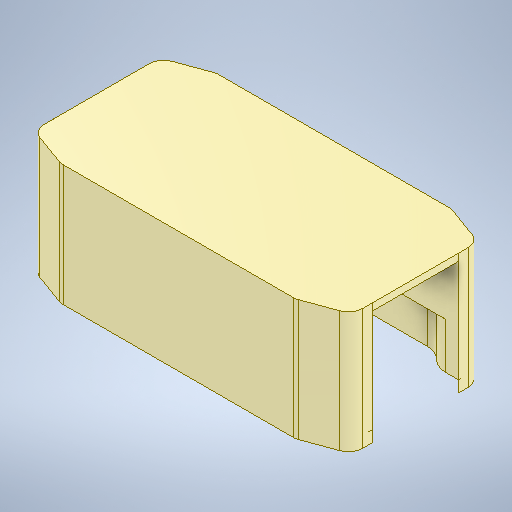
# Autodesk Inventor part: Housing_Upper
Saved by Autodesk Inventor 2025.1 (Build 291241020, 241B)
## iProperties
Created: 2024-09-09
Part Number: Housing_Upper
Material: Nylon 6/6
Document SubType Name: Modeling
Designer: ahorat
Density: 1.13 g/cm^3
Appearance: Nylon 6
Author: ahorat
Autodesk Inventor part; units mm, degrees
ref_plane "YZ Plane" through (0, 0, 0) normal (1, 0, 0) x (0, 1, 0)
ref_plane "XZ Plane" through (0, 0, 0) normal (0, 1, 0) x (-1, 0, 0)
ref_plane "XY Plane" through (0, 0, 0) normal (0, 0, 1) x (1, 0, 0)
sketch "Sketch1" plane through (0, 0, 0) normal (0, 1, 0) x (-1, 0, 0)
  line L0 (22.5664, -5.4388) -> (16.7365, -5.4388)
  arc A0 (16.7365, -5.4388) -> (14.5685, -6.3368) centre (16.7354, -8.502) ccw
  line L1 (14.5685, -6.3368) -> (14.4645, -6.4408)
  arc A1 (12.2965, -7.3388) -> (14.4645, -6.4408) centre (12.2977, -4.2756) ccw
  line L2 (12.2965, -7.3388) -> (-16.1635, -7.3388)
  arc A2 (-18.3315, -6.4408) -> (-16.1635, -7.3388) centre (-16.1646, -4.2756) ccw
  line L3 (-18.3315, -6.4408) -> (-18.4355, -6.3368)
  arc A3 (-18.4355, -6.3368) -> (-20.6023, -5.4388) centre (-20.6023, -8.502) ccw
  line L4 (-20.6023, -5.4388) -> (-22.4336, -5.4388)
  arc A4 (-22.4336, -5.4388) -> (-20.4336, -7.4388) centre (-20.4336, -5.4388) ccw
  line L5 (-20.4336, -7.4388) -> (-20.6024, -7.4388)
  arc A5 (-19.8506, -7.7502) -> (-20.6024, -7.4388) centre (-20.6024, -8.502) ccw
  line L6 (-19.8506, -7.7502) -> (-19.745, -7.8558)
  arc A6 (-19.745, -7.8558) -> (-16.1648, -9.3388) centre (-16.1648, -4.2756) ccw
  line L7 (-16.1648, -9.3388) -> (12.2976, -9.3388)
  arc A7 (12.2976, -9.3388) -> (15.8778, -7.8558) centre (12.2976, -4.2756) ccw
  line L8 (15.8778, -7.8558) -> (15.9834, -7.7502)
  arc A8 (16.7352, -7.4388) -> (15.9834, -7.7502) centre (16.7352, -8.502) ccw
  line L9 (16.7352, -7.4388) -> (20.5664, -7.4388)
  arc A9 (20.5664, -7.4388) -> (22.5664, -5.4388) centre (20.5664, -5.4388) ccw
  line L10 (20.5665, 8.7612) -> (16.7354, 8.7612)
  arc A10 (15.9836, 9.0726) -> (16.7354, 8.7612) centre (16.7354, 9.8244) ccw
  line L11 (15.9836, 9.0726) -> (15.8779, 9.1782)
  arc A11 (15.8779, 9.1782) -> (12.2977, 10.6612) centre (12.2977, 5.598) ccw
  line L12 (12.2977, 10.6612) -> (-16.1646, 10.6612)
  arc A12 (-16.1646, 10.6612) -> (-19.7449, 9.1782) centre (-16.1646, 5.598) ccw
  line L13 (-19.7449, 9.1782) -> (-19.8505, 9.0726)
  arc A13 (-20.6023, 8.7612) -> (-19.8505, 9.0726) centre (-20.6023, 9.8244) ccw
  line L14 (-20.6023, 8.7612) -> (-20.4335, 8.7612)
  arc A14 (-20.4335, 8.7612) -> (-22.4335, 6.7612) centre (-20.4335, 6.7612) ccw
  line L15 (-22.4335, 6.7612) -> (-20.6023, 6.7612)
  arc A15 (-20.6034, 6.7612) -> (-18.436, 7.6592) centre (-20.6029, 9.8244) ccw
  line L16 (-18.436, 7.6592) -> (-18.332, 7.7632)
  arc A16 (-16.164, 8.6612) -> (-18.332, 7.7632) centre (-16.1652, 5.598) ccw
  line L17 (-16.164, 8.6612) -> (12.296, 8.6612)
  arc A17 (14.464, 7.7632) -> (12.296, 8.6612) centre (12.2971, 5.598) ccw
  line L18 (14.464, 7.7632) -> (14.568, 7.6592)
  arc A18 (14.568, 7.6592) -> (16.736, 6.7612) centre (16.7348, 9.8244) ccw
  line L19 (16.736, 6.7612) -> (22.5665, 6.7612)
  arc A19 (21.5662, 6.7612) -> (21.5656, 6.7612) centre (21.5659, 5.7608) ccw
  arc A20 (22.5665, 6.7612) -> (20.5665, 8.7612) centre (20.5665, 6.7612) ccw
  arc A21 (-20.4335, 8.7612) -> (-22.4335, 6.7612) centre (-20.4335, 6.7612) ccw
  line L20 (-20.6023, 8.7612) -> (-20.4335, 8.7612)
  arc A22 (-20.6023, 8.7612) -> (-19.8505, 9.0726) centre (-20.6023, 9.8244) ccw
  line L21 (-19.7449, 9.1782) -> (-19.8505, 9.0726)
  arc A23 (-16.1646, 10.6612) -> (-19.7449, 9.1782) centre (-16.1646, 5.598) ccw
  line L22 (12.2977, 10.6612) -> (-16.1646, 10.6612)
  arc A24 (15.8779, 9.1782) -> (12.2977, 10.6612) centre (12.2977, 5.598) ccw
  line L23 (15.9836, 9.0726) -> (15.8779, 9.1782)
  arc A25 (15.9836, 9.0726) -> (16.7354, 8.7612) centre (16.7354, 9.8244) ccw
  line L24 (20.5665, 8.7612) -> (16.7354, 8.7612)
  arc A26 (22.5665, 6.7612) -> (20.5665, 8.7612) centre (20.5665, 6.7612) ccw
  line L25 (22.5665, 6.7612) -> (22.5665, 8.1075)
  arc A27 (22.5665, 8.1075) -> (21.2506, 9.9869) centre (20.5665, 8.1075) ccw
  line L26 (21.2506, 9.9869) -> (16.9818, 11.5406)
  arc A28 (16.9818, 11.5406) -> (16.2977, 11.6612) centre (16.2977, 9.6612) ccw
  line L27 (16.2977, 11.6612) -> (-16.1646, 11.6612)
  arc A29 (-16.1646, 11.6612) -> (-16.8487, 11.5406) centre (-16.1646, 9.6612) ccw
  line L28 (-16.8487, 11.5406) -> (-21.1175, 9.9869)
  arc A30 (-21.1175, 9.9869) -> (-22.4335, 8.1075) centre (-20.4335, 8.1075) ccw
  line L29 (-22.4335, 8.1075) -> (-22.4335, 6.7612)
  arc A31 (20.5664, -7.4388) -> (22.5664, -5.4388) centre (20.5664, -5.4388) ccw
  line L30 (16.7352, -7.4388) -> (20.5664, -7.4388)
  arc A32 (16.7352, -7.4388) -> (15.9834, -7.7502) centre (16.7352, -8.502) ccw
  line L31 (15.8778, -7.8558) -> (15.9834, -7.7502)
  arc A33 (12.2976, -9.3388) -> (15.8778, -7.8558) centre (12.2976, -4.2756) ccw
  line L32 (-16.1648, -9.3388) -> (12.2976, -9.3388)
  arc A34 (-19.745, -7.8558) -> (-16.1648, -9.3388) centre (-16.1648, -4.2756) ccw
  line L33 (-19.8506, -7.7502) -> (-19.745, -7.8558)
  arc A35 (-19.8506, -7.7502) -> (-20.6024, -7.4388) centre (-20.6024, -8.502) ccw
  line L34 (-20.4336, -7.4388) -> (-20.6024, -7.4388)
  arc A36 (-22.4336, -5.4388) -> (-20.4336, -7.4388) centre (-20.4336, -5.4388) ccw
  line L35 (-22.4336, -5.4388) -> (-22.4336, -6.7851)
  arc A37 (-22.4336, -6.7851) -> (-21.1177, -8.6645) centre (-20.4336, -6.7851) ccw
  line L36 (-21.1177, -8.6645) -> (-16.8488, -10.2182)
  arc A38 (-16.8488, -10.2182) -> (-16.1648, -10.3388) centre (-16.1648, -8.3388) ccw
  line L37 (-16.1648, -10.3388) -> (16.2976, -10.3388)
  arc A39 (16.2976, -10.3388) -> (16.9816, -10.2182) centre (16.2976, -8.3388) ccw
  line L38 (16.9816, -10.2182) -> (21.2504, -8.6645)
  arc A40 (21.2504, -8.6645) -> (22.5664, -6.7851) centre (20.5664, -6.7851) ccw
  line L39 (22.5664, -6.7851) -> (22.5664, -5.4388)
  point P0 (-0.0157, -0.0172)
  point P1 (-21.4334, -5.4388)
  point P2 (-21.4334, -5.4388)
  point P3 (-22.3448, 6.1725)
  point P4 (-21.4334, 6.7612)
  point P5 (22.5666, -5.4399)
  point P6 (-14.0216, -19.3432)
  point P7 (-20.5993, -7.4388)
  point P8 (-22.4334, -5.4388)
  point P9 (-22.4334, 6.7612)
  point P10 (-20.4334, 8.7612)
  point P11 (-20.6017, 8.7612)
  point P12 (20.5666, 8.7612)
  point P13 (22.5666, -5.4388)
  constraints: 84 point on circle, 80 end point, 41 centre point, 6 point on line
extrude "Extrusion1" add sketch "Sketch1" along normal blind 14.5 contours A9 L9 A8 L8 A7 L7 A6 L6 A5 L5 A4 L4 A3 L3 A2 L2 A1 L1 A0 L0 | L39 A40 L38 A39 L37 A38 L36 A37 L35 A4 L5 A5 L6 A6 L7 A7 L8 A8 L9 A9 | A20 L19 A18 L18 A17 L17 A16 L16 A15 L15 A14 L14 A13 L13 A12 L12 A11 L11 A10 L10 | L10 A10 L11 A11 L12 A12 L13 A13 L14 A14 L29 A30 L28 A29 L27 A28 L26 A27 L25 A20
extrude "Extrusion2" add sketch "Sketch1" against normal blind 1.6 contours L39 A40 L38 A39 L37 A38 L36 A37 L35 A4 L5 A5 L6 A6 L7 A7 L8 A8 L9 A9 | L10 A10 L11 A11 L12 A12 L13 A13 L14 A14 L29 A30 L28 A29 L27 A28 L26 A27 L25 A20
sketch "Sketch3" plane through (0, 0, 0) normal (1, 0, 0) x (0, 1, 0)
  line L0 (0, -9.3388) -> (-1.6, -9.3388) projected
  line L1 (-1.4, -9.3388) -> (-1, -8.9388)
  line L2 (-1, -8.9388) -> (-0.6, -9.3388)
  line L3 (0, 10.6612) -> (-1.6, 10.6612) projected
  line L4 (-1.4, 10.6612) -> (-1, 10.2612)
  line L5 (-1, 10.2612) -> (-0.6, 10.6612)
  point P0 (0, 0)
  point P1 (-0.8, 10.6612)
  dimension "d4" = 0.4
  dimension "d6" = 0.4
  dimension "d33" = 1
  dimension "d34" = 1
  constraints: 8 end point, 4 perpendicular, 4 point on line, 1 midpoint
  measures "d4" distance from line of L1.end L0
  measures "d6" vertical distance of point (-0.8, 10.661) L4.end
  measures "d33" horizontal distance of L0.start L1.end
  measures "d34" horizontal distance of L3.start L4.end
extrude "Extrusion3" add sketch "Sketch3" along normal mid plane 8
sketch "Sketch4" plane through (0, 14.5, 0) normal (0, 1, 0) x (1, 0, 0)
  arc A0 (-16.7365, 5.4388) -> (-14.5685, 6.3368) centre (-16.7354, 8.502) ccw projected
  line L0 (-14.5685, 6.3368) -> (-14.4645, 6.4408) projected
  arc A1 (-12.2965, 7.3388) -> (-14.4645, 6.4408) centre (-12.2977, 4.2756) ccw projected
  line L1 (-12.2965, 7.3388) -> (16.1635, 7.3388) projected
  arc A2 (18.3315, 6.4408) -> (16.1635, 7.3388) centre (16.1646, 4.2756) ccw projected
  line L2 (18.3315, 6.4408) -> (18.4355, 6.3368) projected
  arc A3 (18.4355, 6.3368) -> (20.6023, 5.4388) centre (20.6023, 8.502) ccw projected
  line L3 (20.6023, 5.4388) -> (22.4336, 5.4388) projected
  line L4 (22.4336, 5.4388) -> (22.4336, 6.7851) projected
  arc A4 (22.4336, 6.7851) -> (21.1177, 8.6645) centre (20.4336, 6.7851) ccw projected
  line L5 (21.1177, 8.6645) -> (16.8488, 10.2182) projected
  arc A5 (16.8488, 10.2182) -> (16.1648, 10.3388) centre (16.1648, 8.3388) ccw projected
  line L6 (16.1648, 10.3388) -> (-16.2976, 10.3388) projected
  arc A6 (-16.2976, 10.3388) -> (-16.9816, 10.2182) centre (-16.2976, 8.3388) ccw projected
  line L7 (-16.9816, 10.2182) -> (-21.2504, 8.6645) projected
  arc A7 (-21.2504, 8.6645) -> (-22.5664, 6.7851) centre (-20.5664, 6.7851) ccw projected
  line L8 (-22.5664, 6.7851) -> (-22.5664, 5.4388) projected
  line L9 (-22.5664, 5.4388) -> (-16.7365, 5.4388) projected
  arc A8 (-22.5665, -8.1075) -> (-21.2506, -9.9869) centre (-20.5665, -8.1075) ccw projected
  line L10 (-21.2506, -9.9869) -> (-16.9818, -11.5406) projected
  arc A9 (-16.9818, -11.5406) -> (-16.2977, -11.6612) centre (-16.2977, -9.6612) ccw projected
  line L11 (-16.2977, -11.6612) -> (16.1646, -11.6612) projected
  arc A10 (16.1646, -11.6612) -> (16.8487, -11.5406) centre (16.1646, -9.6612) ccw projected
  line L12 (16.8487, -11.5406) -> (21.1175, -9.9869) projected
  arc A11 (21.1175, -9.9869) -> (22.4335, -8.1075) centre (20.4335, -8.1075) ccw projected
  line L13 (22.4335, -8.1075) -> (22.4335, -6.7612) projected
  line L14 (22.4335, -6.7612) -> (20.6023, -6.7612) projected
  arc A12 (20.6023, -6.7612) -> (18.436, -7.6592) centre (20.6029, -9.8244) ccw projected
  line L15 (18.436, -7.6592) -> (18.332, -7.7632) projected
  arc A13 (16.164, -8.6612) -> (18.332, -7.7632) centre (16.1652, -5.598) ccw projected
  line L16 (16.164, -8.6612) -> (-12.296, -8.6612) projected
  arc A14 (-14.464, -7.7632) -> (-12.296, -8.6612) centre (-12.2971, -5.598) ccw projected
  line L17 (-14.464, -7.7632) -> (-14.568, -7.6592) projected
  arc A15 (-14.568, -7.6592) -> (-16.736, -6.7612) centre (-16.7348, -9.8244) ccw projected
  line L18 (-16.736, -6.7612) -> (-22.5665, -6.7612) projected
  line L19 (-22.5665, -6.7612) -> (-22.5665, -8.1075) projected
  line L20 (22.4336, 5.4388) -> (22.4335, -6.7612)
  line L21 (-16.736, -6.7612) -> (-22.5665, -6.7612) projected
  line L22 (-22.5665, -6.7612) -> (-22.5664, 5.4388)
  point P0 (0, 0)
  constraints: 4 end point
extrude "Extrusion4" add sketch "Sketch4" along normal blind 1
sketch "Sketch5" plane through (0, 14.5, 0) normal (0, -1, 0) x (1, 0, 0)
  line L0 (20.6023, -5.4388) -> (22.4336, -5.4388) projected
  line L1 (22.4335, 6.7612) -> (22.4336, -5.4388) projected
  line L2 (22.4335, 6.7612) -> (20.6023, 6.7612) projected
  arc A0 (18.436, 7.6592) -> (20.6023, 6.7612) centre (20.6029, 9.8244) ccw projected
  line L3 (18.436, 7.6592) -> (18.332, 7.7632) projected
  arc A1 (18.332, 7.7632) -> (16.164, 8.6612) centre (16.1652, 5.598) ccw projected
  line L4 (16.164, 8.6612) -> (-12.296, 8.6612) projected
  arc A2 (-12.296, 8.6612) -> (-14.464, 7.7632) centre (-12.2971, 5.598) ccw projected
  line L5 (-14.464, 7.7632) -> (-14.568, 7.6592) projected
  arc A3 (-16.736, 6.7612) -> (-14.568, 7.6592) centre (-16.7348, 9.8244) ccw projected
  line L6 (-16.736, 6.7612) -> (-22.5665, 6.7612) projected
  line L7 (-22.5664, -5.4388) -> (-22.5665, 6.7612) projected
  line L8 (-22.5664, -5.4388) -> (-16.7365, -5.4388) projected
  arc A4 (-14.5685, -6.3368) -> (-16.7365, -5.4388) centre (-16.7354, -8.502) ccw projected
  line L9 (-14.5685, -6.3368) -> (-14.4645, -6.4408) projected
  arc A5 (-14.4645, -6.4408) -> (-12.2965, -7.3388) centre (-12.2977, -4.2756) ccw projected
  line L10 (-12.2965, -7.3388) -> (16.1635, -7.3388) projected
  arc A6 (16.1635, -7.3388) -> (18.3315, -6.4408) centre (16.1646, -4.2756) ccw projected
  line L11 (18.3315, -6.4408) -> (18.4355, -6.3368) projected
  arc A7 (20.6023, -5.4388) -> (18.4355, -6.3368) centre (20.6023, -8.502) ccw projected
  arc A8 (-14.5685, -6.3368) -> (-16.7365, -5.4388) centre (-16.7354, -8.502) ccw projected
  line L12 (-16.7365, -5.4388) -> (-5.9665, -5.4347)
  line L13 (-5.9665, 6.7571) -> (-16.736, 6.7612)
  line L14 (-5.9665, -5.4347) -> (-5.9665, 6.7571)
  point P0 (0, 0)
  point P1 (-22.5665, 0.6612)
  point P2 (-5.9665, 0.6612)
  dimension "d13" = 16.6
  constraints: 6 end point, 3 tangent, 2 midpoint, 1 vertical
  measures "d13" distance of point (-22.566, 0.661) point (-5.966, 0.661)
extrude "Extrusion5" add sketch "Sketch5" along normal blind 3.6 contours L8 L7 L6 L13 L14 L12
sketch "Sketch6" plane through (0, 14.5, 0) normal (0, -1, 0) x (1, 0, 0)
  line L0 (-16.736, 6.7612) -> (-5.9665, 6.7571) projected
  line L1 (-5.9665, 6.7571) -> (-5.9665, -5.4347) projected
  line L2 (-5.9665, -5.4347) -> (-16.7365, -5.4388) projected
  arc A0 (-14.5685, -6.3368) -> (-16.7365, -5.4388) centre (-16.7354, -8.502) ccw projected
  line L3 (-14.5685, -6.3368) -> (-14.4645, -6.4408) projected
  arc A1 (-14.4645, -6.4408) -> (-12.2965, -7.3388) centre (-12.2977, -4.2756) ccw projected
  line L4 (-12.2965, -7.3388) -> (16.1635, -7.3388) projected
  arc A2 (16.1635, -7.3388) -> (18.3315, -6.4408) centre (16.1646, -4.2756) ccw projected
  line L5 (18.3315, -6.4408) -> (18.4355, -6.3368) projected
  arc A3 (20.6023, -5.4388) -> (18.4355, -6.3368) centre (20.6023, -8.502) ccw projected
  line L6 (20.6023, -5.4388) -> (22.4336, -5.4388) projected
  line L7 (22.4335, 6.7612) -> (22.4336, -5.4388) projected
  line L8 (22.4335, 6.7612) -> (20.6023, 6.7612) projected
  arc A4 (18.436, 7.6592) -> (20.6023, 6.7612) centre (20.6029, 9.8244) ccw projected
  line L9 (18.436, 7.6592) -> (18.332, 7.7632) projected
  arc A5 (18.332, 7.7632) -> (16.164, 8.6612) centre (16.1652, 5.598) ccw projected
  line L10 (16.164, 8.6612) -> (-12.296, 8.6612) projected
  arc A6 (-12.296, 8.6612) -> (-14.464, 7.7632) centre (-12.2971, 5.598) ccw projected
  line L11 (-14.464, 7.7632) -> (-14.568, 7.6592) projected
  arc A7 (-16.736, 6.7612) -> (-14.568, 7.6592) centre (-16.7348, 9.8244) ccw projected
  line L12 (22.4335, 6.7612) -> (22.4336, -5.4388) projected
  line L13 (22.4336, -5.4388) -> (8.8335, -5.4388)
  line L14 (8.8335, -5.4388) -> (8.8335, 6.7612)
  line L15 (8.8335, 6.7612) -> (22.4335, 6.7612)
  line L16 (-12.2965, -7.3388) -> (16.1635, -7.3388) projected
  line L17 (16.164, 8.6612) -> (-12.296, 8.6612) projected
  line L18 (-3.9665, -7.3388) -> (6.8335, -7.3388)
  line L19 (6.8335, -7.3388) -> (6.8335, 8.6612)
  line L20 (6.8335, 8.6612) -> (-3.9665, 8.6612)
  line L21 (-3.9665, 8.6612) -> (-3.9665, -7.3388)
  point P0 (0, 0)
  point P1 (8.8335, 0.6612)
  point P2 (20.6023, -5.4388)
  point P3 (-3.9665, 8.6612)
  point P4 (6.8335, -7.3388)
  dimension "d16" = 13.6
  dimension "d19" = 2
  dimension "d20" = 2
  constraints: 14 end point, 3 horizontal, 2 parallel, 2 perpendicular, 2 point on line, 1 midpoint
  measures "d16" distance from line of L7 point (8.834, 0.661)
  measures "d19" distance between parallel lines of L1 L21
  measures "d20" distance between parallel lines of L14 L19
extrude "Extrusion6" add sketch "Sketch6" along normal blind 8 contours A7 L11 A6 L10 L21 L4 A1 L3 A0 L2 L1 L0 | L10 A5 L9 A4 L15 L14 L13 A3 L5 A2 L4 L19
equation "\"d6\" = d4"
equation "\"d34\" = d33"
body "Solid1"
